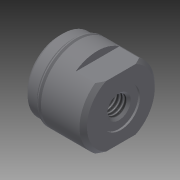
# Autodesk Inventor part: 02R00_NR_rear_head
Saved by Autodesk Inventor 2013 (Build 170138000, 138)
## iProperties
Category: PARTsolutions
Company: BIMBA
Created: 2013-01-26
Part Number: 02R00_NR_rear_head
Material: Generic
Catalog Web Link: www.cadenas.de
Description: NR Rear Head-Original Line Cylinders
Vendor: BIMBA
Document SubType Name: Modeling
Designer: actoennies
Manufacturer: BIMBA
Density: 1 g/cm^3
Mass: 2.00741 g
Surface Area: 11.8707 cm^2
Volume: 2.00741 cm^3
PSOL_IDENT_0: {\\10.0.0.242\data_v9\23d-libs\bimba\bimba\bimba_imperial\bimba_full_line\original_line_cylinders\no
PSOL_IDENT_1: n_rotating_air_cylinders\non_rot_rear_head.prj},200 {VTYP=3D},{NB=02R00_NR_rear_head},{LINA=02R00_NR
PSOL_IDENT_2: _rear_head},{NN=NR Rear Head},{DATE=29.09.2011 07:02:13},{GEOMDATE=20.04.2011 07:00:00},{VERSION=},{
PSOL_IDENT_3: LINEID=30},{LINESUBID=-1},{WBVAR=MNT,ACTING,Q,Y,K}  {NB=02R00_NR_rear_head},{LINA=02R00_NR_rear_head
PSOL_IDENT_4: },{KT=DUMMY},{PN=02R00},{BORE=0.56250},{BOREPN=02},{MNT=},{MNTALG='' , 'Front Nose' , 'P' , 'Rear Pi
PSOL_IDENT_5: vot'},{ACTING=R},{ACTINGALG= '' , 'Single Acting' , 'R' , 'Reverse/Double Acting' },{DER=},{DERALG=
PSOL_IDENT_6: '' , 'Standard' },{Q=},{T1=},{T2=},{T3=},{T4=},{TRIM=0},{Y=},{K=},{KALG= '', 'without K', 'K', 'with
PSOL_IDENT_7: K' },{A1=0.5000},{A1N=0.5000},{A1P=0.9690},{A1B=0.0000},{A1S=0.0000},{A2=0.157},{A2N=0.1570},{A3=0.
PSOL_IDENT_8: 0250},{D1=0.6095},{D1N=0.6095},{D1P=0.6150},{D1B=0.0000},{D2=0.5725},{C1=0.0300},{C2=0.0300},{NDM=0.
PSOL_IDENT_9: 1900},{TAB=UNF},{NDMDP=0.2000},{D3=0.1600},{A4=0.1900},{A5=0.4950},{D4=0.0000},{A6=0.0000},{A7=0.375
PSOL_IDENT_10: 0},{A8=0.0000},{D5=0.0000},{D6=0.1540},{A9=0.4400},{NDM2=0.4375},{TAB2=UNF},{C11=0.0300},{C22=0.0000
PSOL_IDENT_11: },{C33=0.0300},{C44=0.0300},{A10=0.3070},{A11=0.0000},{NDM3=0.1900},{NDM3N=0.1900},{NDM3B=0.0000},{T
PSOL_IDENT_12: AB3=UNF},{TAB3N=UNF},{TAB3B=-},{A12=0.406},{A12N=0.4060},{A12B=0.0000},{A13=0.7810},{D7=0.1570},{D71
PSOL_IDENT_13: =0.15700000},{D72=0.15700000},{D77=0.157},{D8=0.4355},{D88=0.43550000},{A14=0.0620},{A15=0.0775},{D9
PSOL_IDENT_14: =0.3600},{R1=0.0315},{X1=0.0000},{X2=0.0000},{CX=0.0000},{CC=0.0000},{CON=0},{S1=0.0000},{DB=0.0000}
PSOL_IDENT_15: ,{X1B=0.0000},{X2B=0.0000},{A8B=0.0000},{A9B=0.0000},{MODEL=1},{NDM4=0.0000},{TAB4=-},{NDM4DP=0.0000
PSOL_IDENT_16: },{BC=0.0000},{B1=0.0000},{B2=0.0000},{B3=0.0000},{ON=0},{ON2=1},{G1=0.0000},{G2=0.0000},{G3=0.0000}
PSOL_IDENT_17: ,{G4=0.0000},{GD=0},{GD1=0.00000000},{GD2=0.00000000},{G5=0.0000},{G6=0.0000},{RON=0},{H1=0.0000},{H
PSOL_IDENT_18: 2=0.0000},{H3=0.0000},{H4=0.0000},{H5=0.0000},{H6=0.0000},{F=0.0000},{PNUT=0.0000},{CUSH=0},{CC11=0.
PSOL_IDENT_19: 0000},{CC22=0.0000},{CC33=0.0000},{CC44=0.0000},{CC55=0.0000},{CD1=0.0000},{CD2=0.0000},{CD3=0.0000}
PSOL_IDENT_20: ,{CNDM3=0.0000},{CTAB3=0.0000},{OLEN=0.5000},{OD=0.2185}
CNS_NT: Original Line Cylinders
CNS_NB: 02R00_NR_rear_head
CNS_NBSYN: $PN._NR_rear_head
CNS_LINA: 02R00_NR_rear_head
CNS_PN: 02R00
CNS_BORE: 0.56250
CNS_BOREPN: 02
CNS_MNT: Front Nose
CNS_MNTALG: '' , 'Front Nose' , 'P' , 'Rear Pivot'
CNS_ACTING: Reverse/Double Acting
CNS_ACTINGALG: '' , 'Single Acting' , 'R' , 'Reverse/Double Acting'
CNS_DERALG: '' , 'Standard'
CNS_Q: Without Side Ported Rear Head
CNS_TRIM: 0.000
CNS_Y: without Pivot Bushing
CNS_K: without K
CNS_KALG: '', 'without K', 'K', 'with K'
CNS_A1: 0.5000
CNS_A1N: 0.5000
CNS_A1P: 0.9690
CNS_A1B: 0.0000
CNS_A1S: 0.0000
CNS_A2: 0.157
CNS_A2N: 0.1570
CNS_A3: 0.0250
CNS_D1: 0.6095
CNS_D1N: 0.6095
CNS_D1P: 0.6150
CNS_D1B: 0.0000
CNS_D2: 0.5725
CNS_C1: 0.0300
CNS_C2: 0.0300
CNS_NDM: 0.1900
CNS_TAB: UNF
CNS_NDMDP: 0.2000
CNS_D3: 0.1600
CNS_A4: 0.1900
CNS_A5: 0.4950
CNS_D4: 0.0000
CNS_A6: 0.0000
CNS_A7: 0.3750
CNS_A8: 0.0000
CNS_D5: 0.0000
CNS_D6: 0.1540
CNS_A9: 0.4400
CNS_NDM2: 0.4375
CNS_TAB2: UNF
CNS_C11: 0.0300
CNS_C22: 0.0000
CNS_C33: 0.0300
CNS_C44: 0.0300
CNS_A10: 0.3070
CNS_A11: 0.0000
CNS_NDM3: 0.1900
CNS_NDM3N: 0.1900
CNS_NDM3B: 0.0000
CNS_TAB3: UNF
CNS_TAB3N: UNF
CNS_TAB3B: -
CNS_A12: 0.406
CNS_A12N: 0.4060
CNS_A12B: 0.0000
CNS_A13: 0.7810
CNS_D7: 0.1570
CNS_D71: 0.15700000
CNS_D72: 0.15700000
CNS_D77: 0.157
CNS_D8: 0.4355
CNS_D88: 0.43550000
CNS_A14: 0.0620
CNS_A15: 0.0775
CNS_D9: 0.3600
CNS_R1: 0.0315
CNS_X1: 0.0000
CNS_X2: 0.0000
CNS_CX: 0.0000
CNS_CC: 0.0000
CNS_CON: 0
CNS_S1: 0.0000
CNS_DB: 0.0000
CNS_X1B: 0.0000
CNS_X2B: 0.0000
CNS_A8B: 0.0000
CNS_A9B: 0.0000
CNS_MODEL: 1
CNS_NDM4: 0.0000
CNS_TAB4: -
CNS_NDM4DP: 0.0000
CNS_BC: 0.0000
CNS_B1: 0.0000
CNS_B2: 0.0000
CNS_B3: 0.0000
CNS_ON: 0
CNS_ON2: 1
CNS_G1: 0.0000
CNS_G2: 0.0000
CNS_G3: 0.0000
CNS_G4: 0.0000
CNS_GD: 0.000
CNS_GD1: 0.00000000
CNS_GD2: 0.00000000
CNS_G5: 0.0000
CNS_G6: 0.0000
CNS_RON: 0
CNS_H1: 0.0000
CNS_H2: 0.0000
CNS_H3: 0.0000
CNS_H4: 0.0000
CNS_H5: 0.0000
CNS_H6: 0.0000
CNS_F: 0.0000
CNS_PNUT: 0.0000
CNS_CUSH: 0.000
CNS_CC11: 0.0000
CNS_CC22: 0.0000
CNS_CC33: 0.0000
CNS_CC44: 0.0000
CNS_CC55: 0.0000
CNS_CD1: 0.0000
CNS_CD2: 0.0000
CNS_CD3: 0.0000
CNS_CNDM3: 0.0000
CNS_CTAB3: 0.0000
CNS_OLEN: 0.5000
CNS_OD: 0.2185
SUPPLIER: BIMBA
ARTICLENO: 02R00_NR_rear_head
BOMINFO: 02R00_NR_rear_head
CREATOR: CADENAS GmbH
Title: 02R00_NR_rear_head
Author: Cadenas PARTsolutions
Comments: Original Line Cylinders
Autodesk Inventor part; units mm, degrees
sketch "Sketch_1" plane through (0, 0, 0) normal (0, 0, 1) x (1, 0, 0)
  line L0 (12.7, 0) -> (0, 0)
  line L1 (0, 0) -> (0, 6.5088)
  line L2 (0, 6.5088) -> (0.762, 7.2708)
  line L3 (0.762, 7.2708) -> (2.7178, 7.2708)
  line L4 (2.7178, 7.2708) -> (3.3528, 6.6357)
  line L5 (3.3528, 6.6357) -> (3.9878, 6.6357)
  line L6 (3.9878, 6.6357) -> (3.9878, 7.7407)
  line L7 (3.9878, 7.7407) -> (11.938, 7.7407)
  line L8 (11.938, 7.7407) -> (12.7, 6.9787)
  line L9 (12.7, 6.9787) -> (12.7, 0)
  line L10 (12.7, 0) -> (0, 0)
  constraints: 22 end point
revolve "Revolution1" add sketch "Sketch_1" angle 360 about axis through (12.7, 0, 0) along (1, 0, 0)
sketch "Sketch2" plane through (12.7, 0, 0) normal (1, 0, 0) x (0, 0, -1)
  point P0 (0, 0)
hole "Drilling 1" at (12.7, 0, 0) direction (-1, 0, 0) diameter 7.9248 depth 0.381
sketch "Sketch3" plane through (12.319, 0, 0) normal (1, 0, 0) x (0, 0, -1)
  point P0 (0, 0)
hole "Drilling 2" at (12.319, 0, 0) direction (-1, 0, 0) diameter 3.9624 depth 12.319 countersink diameter 4.826 countersink angle 90 thread size "10-32 UNF" class "2B" standard "ANSI Unified Screw Threads"
sketch "Sketch_5" plane through (12.7, 0, 0) normal (1, 0, 0) x (0, 0, -1)
  line L0 (-30.9626, 15.4813) -> (-30.9626, -15.4813)
  line L1 (-30.9626, -15.4813) -> (30.9626, -15.4813)
  line L2 (30.9626, -15.4813) -> (30.9626, 15.4813)
  line L3 (30.9626, 15.4813) -> (-30.9626, 15.4813)
  line L4 (-15.4813, 6.2865) -> (-15.4813, -6.2865)
  line L5 (-15.4813, -6.2865) -> (15.4813, -6.2865)
  line L6 (15.4813, -6.2865) -> (15.4813, 6.2865)
  line L7 (15.4813, 6.2865) -> (-15.4813, 6.2865)
  constraints: 16 end point
extrude "Extrusion1" cut sketch "Sketch_5" against normal blind 4.826
sketch "Sketch_24" plane through (0, 0, 0) normal (0, 0, 1) x (1, 0, 0)
  line L0 (3.9878, 0) -> (3.3528, 0)
  line L1 (3.2301, 7.6565) -> (3.8708, 7.0158)
  arc A0 (3.8708, 6.8362) -> (3.8708, 7.0158) centre (3.781, 6.926) ccw
  line L2 (3.8708, 6.8362) -> (3.6703, 6.6357)
  line L3 (3.6703, 6.6357) -> (3.3528, 6.6357)
  line L4 (3.3528, 6.6357) -> (3.3528, 6.3818)
  line L5 (3.3528, 6.3818) -> (3.9878, 6.3818)
  line L6 (3.9878, 6.3818) -> (3.9878, 7.1861)
  line L7 (3.9878, 7.1861) -> (3.4333, 7.7407)
  line L8 (3.4333, 7.7407) -> (3.2301, 7.7407)
  line L9 (3.2301, 7.7407) -> (3.2301, 7.6565)
  constraints: 20 end point, 2 point on circle, 1 centre point
revolve "Revolution2" add sketch "Sketch_24" angle 360 about axis through (3.9878, 0, 0) along (1, 0, 0)
ref_plane "cut1_XY" through (12.7, 6.2865, 0) normal (1, 0, 0) x (0, 0, -1)
ref_plane "cut1_YZ" through (12.7, 6.2865, 0) normal (0, 0, -1) x (0, 1, 0)
ref_plane "cut1_ZX" through (12.7, 6.2865, 0) normal (0, 1, 0) x (1, 0, 0)
ref_plane "cut2_XY" through (12.7, -6.2865, 0) normal (1, 0, 0) x (0, 0, -1)
ref_plane "cut2_YZ" through (12.7, -6.2865, 0) normal (0, 0, -1) x (0, 1, 0)
ref_plane "cut2_ZX" through (12.7, -6.2865, 0) normal (0, 1, 0) x (1, 0, 0)
ref_plane "to_tube_XY" through (3.3528, 0, 0) normal (1, 0, 0) x (0, 0, -1)
ref_plane "to_tube_YZ" through (3.3528, 0, 0) normal (0, 0, -1) x (0, 1, 0)
ref_plane "to_tube_ZX" through (3.3528, 0, 0) normal (0, 1, 0) x (1, 0, 0)
ref_plane "lovra_XY" through (12.7, 0, 0) normal (1, 0, 0) x (0, 1, 0)
ref_plane "lovra_YZ" through (12.7, 0, 0) normal (0, 1, 0) x (0, 0, 1)
ref_plane "lovra_ZX" through (12.7, 0, 0) normal (0, 0, 1) x (1, 0, 0)
ref_plane "to_nut_XY" through (0, 0, 0) normal (1, 0, 0) x (0, 0, -1)
ref_plane "to_nut_YZ" through (0, 0, 0) normal (0, 0, -1) x (0, 1, 0)
ref_plane "to_nut_ZX" through (0, 0, 0) normal (0, 1, 0) x (1, 0, 0)
ref_plane "lovra1_XY" through (7.874, 0, 0) normal (1, 0, 0) x (0, 0, -1)
ref_plane "lovra1_YZ" through (7.874, 0, 0) normal (0, 0, -1) x (0, 1, 0)
ref_plane "lovra1_ZX" through (7.874, 0, 0) normal (0, 1, 0) x (1, 0, 0)
ref_plane "lovra2_XY" through (7.874, 6.2865, 0) normal (1, 0, 0) x (0, 0, -1)
ref_plane "lovra2_YZ" through (7.874, 6.2865, 0) normal (0, 0, -1) x (0, 1, 0)
ref_plane "lovra2_ZX" through (7.874, 6.2865, 0) normal (0, 1, 0) x (1, 0, 0)
ref_plane "lovra3_XY" through (7.874, -6.2865, 0) normal (1, 0, 0) x (0, 0, -1)
ref_plane "lovra3_YZ" through (7.874, -6.2865, 0) normal (0, 0, -1) x (0, 1, 0)
ref_plane "lovra3_ZX" through (7.874, -6.2865, 0) normal (0, 1, 0) x (1, 0, 0)
ref_plane "olen_XY" through (12.7, 0, 0) normal (1, 0, 0) x (0, 0, -1)
ref_plane "olen_YZ" through (12.7, 0, 0) normal (0, 0, -1) x (0, 1, 0)
ref_plane "olen_ZX" through (12.7, 0, 0) normal (0, 1, 0) x (1, 0, 0)
ref_plane "cutf1_XY" through (12.7, 7.7407, 0) normal (0, 0, 1) x (1, 0, 0)
ref_plane "cutf1_YZ" through (12.7, 7.7407, 0) normal (1, 0, 0) x (0, 1, 0)
ref_plane "cutf1_ZX" through (12.7, 7.7407, 0) normal (0, 1, 0) x (0, 0, 1)
ref_plane "cutf2_XY" through (7.874, 7.7407, 0) normal (0, 0, 1) x (1, 0, 0)
ref_plane "cutf2_YZ" through (7.874, 7.7407, 0) normal (1, 0, 0) x (0, 1, 0)
ref_plane "cutf2_ZX" through (7.874, 7.7407, 0) normal (0, 1, 0) x (0, 0, 1)
ref_plane "lovra21_XY" through (0, 0, 5.2705) normal (1, 0, 0) x (0, 0, -1)
ref_plane "lovra21_YZ" through (0, 0, 5.2705) normal (0, 0, -1) x (0, 1, 0)
ref_plane "lovra21_ZX" through (0, 0, 5.2705) normal (0, 1, 0) x (1, 0, 0)
ref_plane "lovra22_XY" through (0, 0, -5.2705) normal (1, 0, 0) x (0, 0, -1)
ref_plane "lovra22_YZ" through (0, 0, -5.2705) normal (0, 0, -1) x (0, 1, 0)
ref_plane "lovra22_ZX" through (0, 0, -5.2705) normal (0, 1, 0) x (1, 0, 0)
ref_plane "to_pin_XY" through (19.8374, 0, 0) normal (0, 0, 1) x (1, 0, 0)
ref_plane "to_pin_YZ" through (19.8374, 0, 0) normal (1, 0, 0) x (0, 1, 0)
ref_plane "to_pin_ZX" through (19.8374, 0, 0) normal (0, 1, 0) x (0, 0, 1)
ref_plane "mbr_XY" through (13.5128, 0, 0) normal (1, 0, 0) x (0, 0, -1)
ref_plane "mbr_YZ" through (13.5128, 0, 0) normal (0, 0, -1) x (0, 1, 0)
ref_plane "mbr_ZX" through (13.5128, 0, 0) normal (0, 1, 0) x (1, 0, 0)
ref_plane "to_nut1_XY" through (15.0876, 0, 0) normal (1, 0, 0) x (0, 0, -1)
ref_plane "to_nut1_YZ" through (15.0876, 0, 0) normal (0, 0, -1) x (0, 1, 0)
ref_plane "to_nut1_ZX" through (15.0876, 0, 0) normal (0, 1, 0) x (1, 0, 0)
body "Solid1"
